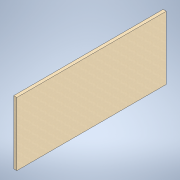
# Autodesk Inventor part: PlatteAußenGross
Saved by Autodesk Inventor 2020.3 (Build 243373000, 373)
## iProperties
Created: 2021-02-12
Part Number: PlatteAußenGross
Material: Generisch
Document SubType Name: Modeling
Designer: Stefan
Density: 1 g/cm^3
Appearance: Pappel
Author: Stefan
Autodesk Inventor part; units mm, degrees
(part 1 of 7)
ref_plane "YZ Plane" through (0, 0, 0) normal (1, 0, 0) x (0, 1, 0)
ref_plane "XZ Plane" through (0, 0, 0) normal (0, 1, 0) x (-1, 0, 0)
ref_plane "XY Plane" through (0, 0, 0) normal (0, 0, 1) x (1, 0, 0)
sketch "Skizze1" plane through (0, 0, 0) normal (1, 0, 0) x (0, 1, 0)
  line L0 (-106.6709, 345.5) -> (93.3291, 345.5)
  line L1 (93.3291, 345.5) -> (93.3291, -126.054)
  line L2 (93.3291, -126.054) -> (-106.6709, -126.054)
  line L3 (-106.6709, -126.054) -> (-106.6709, 345.5)
  point P0 (0, 0)
  dimension "d0" = 200
  dimension "d1" = 471.554
  constraints: 8 end point, 2 parallel, 1 horizontal, 1 perpendicular
  measures "d0" distance of L1.end L2.end
  measures "d1" distance of L0.end L1.end
extrude "Extrusion1" add sketch "Skizze1" along normal blind 10
sketch "Skizze2" plane through (10, 0, 0) normal (1, 0, 0) x (0, 0, -1)
  line L0 (-283.1268, 2.1114) -> (-286.566, 2.1114)
  line L1 (-286.566, 2.1114) -> (-286.566, 4.3601)
  line L2 (-286.566, 4.3601) -> (-286.566, 6.6088)
  line L3 (-286.566, 6.6088) -> (-285.7723, 6.6088)
  line L4 (-285.7723, 6.6088) -> (-285.5154, 6.605)
  line L5 (-285.5154, 6.605) -> (-285.3209, 6.584)
  line L6 (-285.3209, 6.584) -> (-285.1802, 6.5313)
  line L7 (-285.1802, 6.5313) -> (-285.0845, 6.4324)
  line L8 (-285.0845, 6.4324) -> (-285.0252, 6.2729)
  line L9 (-285.0252, 6.2729) -> (-284.9935, 6.0383)
  line L10 (-284.9935, 6.0383) -> (-284.9854, 5.8883)
  line L11 (-284.9854, 5.8883) -> (-284.9809, 5.7142)
  line L12 (-284.9809, 5.7142) -> (-284.9791, 5.514)
  line L13 (-284.9791, 5.514) -> (-284.9787, 5.286)
  line L14 (-284.9787, 5.286) -> (-284.9738, 4.9489)
  line L15 (-284.9738, 4.9489) -> (-284.9586, 4.6676)
  line L16 (-284.9586, 4.6676) -> (-284.9322, 4.4386)
  line L17 (-284.9322, 4.4386) -> (-284.8934, 4.2586)
  line L18 (-284.8934, 4.2586) -> (-284.8415, 4.1244)
  line L19 (-284.8415, 4.1244) -> (-284.7755, 4.0327)
  line L20 (-284.7755, 4.0327) -> (-284.6943, 3.9801)
  line L21 (-284.6943, 3.9801) -> (-284.5971, 3.9632)
  line L22 (-284.5971, 3.9632) -> (-284.5048, 3.9802)
  line L23 (-284.5048, 3.9802) -> (-284.4229, 4.0313)
  line L24 (-284.4229, 4.0313) -> (-284.351, 4.1172)
  line L25 (-284.351, 4.1172) -> (-284.2889, 4.2383)
  line L26 (-284.2889, 4.2383) -> (-284.2364, 4.3954)
  line L27 (-284.2364, 4.3954) -> (-284.1933, 4.589)
  line L28 (-284.1933, 4.589) -> (-284.1592, 4.8195)
  line L29 (-284.1592, 4.8195) -> (-284.1341, 5.0876)
  line L30 (-284.1341, 5.0876) -> (-284.1051, 5.4387)
  line L31 (-284.1051, 5.4387) -> (-284.0699, 5.7083)
  line L32 (-284.0699, 5.7083) -> (-284.02, 5.9069)
  line L33 (-284.02, 5.9069) -> (-283.9472, 6.0453)
  line L34 (-283.9472, 6.0453) -> (-283.843, 6.1343)
  line L35 (-283.843, 6.1343) -> (-283.6992, 6.1846)
  line L36 (-283.6992, 6.1846) -> (-283.5073, 6.2069)
  line L37 (-283.5073, 6.2069) -> (-283.2591, 6.2119)
  line L38 (-283.2591, 6.2119) -> (-283.0108, 6.2069)
  line L39 (-283.0108, 6.2069) -> (-282.819, 6.1846)
  line L40 (-282.819, 6.1846) -> (-282.6752, 6.1343)
  line L41 (-282.6752, 6.1343) -> (-282.571, 6.0453)
  line L42 (-282.571, 6.0453) -> (-282.4982, 5.9069)
  line L43 (-282.4982, 5.9069) -> (-282.4483, 5.7083)
  line L44 (-282.4483, 5.7083) -> (-282.4131, 5.4387)
  line L45 (-282.4131, 5.4387) -> (-282.3841, 5.0876)
  line L46 (-282.3841, 5.0876) -> (-282.359, 4.8195)
  line L47 (-282.359, 4.8195) -> (-282.3249, 4.589)
  line L48 (-282.3249, 4.589) -> (-282.2818, 4.3954)
  line L49 (-282.2818, 4.3954) -> (-282.2293, 4.2383)
  line L50 (-282.2293, 4.2383) -> (-282.1672, 4.1172)
  line L51 (-282.1672, 4.1172) -> (-282.0953, 4.0313)
  line L52 (-282.0953, 4.0313) -> (-282.0134, 3.9802)
  line L53 (-282.0134, 3.9802) -> (-281.9211, 3.9632)
  line L54 (-281.9211, 3.9632) -> (-281.8239, 3.9801)
  line L55 (-281.8239, 3.9801) -> (-281.7427, 4.0327)
  line L56 (-281.7427, 4.0327) -> (-281.6767, 4.1244)
  line L57 (-281.6767, 4.1244) -> (-281.6247, 4.2586)
  line L58 (-281.6247, 4.2586) -> (-281.586, 4.4386)
  line L59 (-281.586, 4.4386) -> (-281.5596, 4.6676)
  line L60 (-281.5596, 4.6676) -> (-281.5444, 4.9489)
  line L61 (-281.5444, 4.9489) -> (-281.5395, 5.286)
  line L62 (-281.5395, 5.286) -> (-281.5395, 6.6088)
  line L63 (-281.5395, 6.6088) -> (-280.6136, 6.6088)
  line L64 (-280.6136, 6.6088) -> (-279.6877, 6.6088)
  line L65 (-279.6877, 6.6088) -> (-279.6877, 4.3601)
  line L66 (-279.6877, 4.3601) -> (-279.6877, 2.1114)
  line L67 (-279.6877, 2.1114) -> (-283.1268, 2.1114)
  line L68 (-282.3332, -54.5023) -> (-284.9787, -54.5023)
  line L69 (-284.9787, -54.5023) -> (-284.9787, -55.4282)
  line L70 (-284.9787, -55.4282) -> (-284.9828, -55.7128)
  line L71 (-284.9828, -55.7128) -> (-284.9999, -55.9325)
  line L72 (-284.9999, -55.9325) -> (-285.0371, -56.0958)
  line L73 (-285.0371, -56.0958) -> (-285.1015, -56.2109)
  line L74 (-285.1015, -56.2109) -> (-285.2001, -56.2859)
  line L75 (-285.2001, -56.2859) -> (-285.3401, -56.3293)
  line L76 (-285.3401, -56.3293) -> (-285.5284, -56.3493)
  line L77 (-285.5284, -56.3493) -> (-285.7723, -56.3542)
  line L78 (-285.7723, -56.3542) -> (-286.566, -56.3542)
  line L79 (-286.566, -56.3542) -> (-286.566, -53.5764)
  line L80 (-286.566, -53.5764) -> (-286.566, -50.7986)
  line L81 (-286.566, -50.7986) -> (-285.7723, -50.7986)
  line L82 (-285.7723, -50.7986) -> (-285.5284, -50.8034)
  line L83 (-285.5284, -50.8034) -> (-285.3401, -50.8234)
  line L84 (-285.3401, -50.8234) -> (-285.2001, -50.8668)
  line L85 (-285.2001, -50.8668) -> (-285.1015, -50.9419)
  line L86 (-285.1015, -50.9419) -> (-285.0371, -51.0569)
  line L87 (-285.0371, -51.0569) -> (-284.9999, -51.2202)
  line L88 (-284.9999, -51.2202) -> (-284.9828, -51.44)
  line L89 (-284.9828, -51.44) -> (-284.9787, -51.7245)
  line L90 (-284.9787, -51.7245) -> (-284.9787, -52.6504)
  line L91 (-284.9787, -52.6504) -> (-282.3332, -52.6504)
  line L92 (-282.3332, -52.6504) -> (-279.6877, -52.6504)
  line L93 (-279.6877, -52.6504) -> (-279.6877, -53.5764)
  line L94 (-279.6877, -53.5764) -> (-279.6877, -54.5023)
  line L95 (-279.6877, -54.5023) -> (-282.3332, -54.5023)
  line L96 (-282.3332, -2.915) -> (-284.9787, -2.915)
  line L97 (-284.9787, -2.915) -> (-284.9787, -3.7087)
  line L98 (-284.9787, -3.7087) -> (-284.9838, -3.9454)
  line L99 (-284.9838, -3.9454) -> (-285.0035, -4.1303)
  line L100 (-285.0035, -4.1303) -> (-285.0438, -4.2698)
  line L101 (-285.0438, -4.2698) -> (-285.1109, -4.3701)
  line L102 (-285.1109, -4.3701) -> (-285.2112, -4.4373)
  line L103 (-285.2112, -4.4373) -> (-285.3507, -4.4775)
  line L104 (-285.3507, -4.4775) -> (-285.5357, -4.4972)
  line L105 (-285.5357, -4.4972) -> (-285.7723, -4.5023)
  line L106 (-285.7723, -4.5023) -> (-286.566, -4.5023)
  line L107 (-286.566, -4.5023) -> (-286.566, -1.8569)
  line L108 (-286.566, -1.8569) -> (-286.566, 0.7887)
  line L109 (-286.566, 0.7887) -> (-285.7723, 0.7887)
  line L110 (-285.7723, 0.7887) -> (-285.5284, 0.7838)
  line L111 (-285.5284, 0.7838) -> (-285.3401, 0.7639)
  line L112 (-285.3401, 0.7639) -> (-285.2001, 0.7204)
  line L113 (-285.2001, 0.7204) -> (-285.1015, 0.6454)
  line L114 (-285.1015, 0.6454) -> (-285.0371, 0.5303)
  line L115 (-285.0371, 0.5303) -> (-284.9999, 0.367)
  line L116 (-284.9999, 0.367) -> (-284.9828, 0.1473)
  line L117 (-284.9828, 0.1473) -> (-284.9787, -0.1373)
  line L118 (-284.9787, -0.1373) -> (-284.9787, -1.0632)
  line L119 (-284.9787, -1.0632) -> (-282.3332, -1.0632)
  line L120 (-282.3332, -1.0632) -> (-279.6877, -1.0632)
  line L121 (-279.6877, -1.0632) -> (-279.6877, -1.9891)
  line L122 (-279.6877, -1.9891) -> (-279.6877, -2.915)
  line L123 (-279.6877, -2.915) -> (-282.3332, -2.915)
  line L124 (-283.1268, -23.2854) -> (-286.566, -23.2854)
  line L125 (-286.566, -23.2854) -> (-286.566, -21.337)
  line L126 (-286.566, -21.337) -> (-286.5595, -20.8821)
  line L127 (-286.5595, -20.8821) -> (-286.5395, -20.4663)
  line L128 (-286.5395, -20.4663) -> (-286.5052, -20.0882)
  line L129 (-286.5052, -20.0882) -> (-286.4555, -19.7464)
  line L130 (-286.4555, -19.7464) -> (-286.3897, -19.4396)
  line L131 (-286.3897, -19.4396) -> (-286.3068, -19.1665)
  line L132 (-286.3068, -19.1665) -> (-286.2059, -18.9258)
  line L133 (-286.2059, -18.9258) -> (-286.0863, -18.7161)
  line L134 (-286.0863, -18.7161) -> (-285.9469, -18.536)
  line L135 (-285.9469, -18.536) -> (-285.7869, -18.3843)
  line L136 (-285.7869, -18.3843) -> (-285.6053, -18.2596)
  line L137 (-285.6053, -18.2596) -> (-285.4014, -18.1606)
  line L138 (-285.4014, -18.1606) -> (-285.1743, -18.0859)
  line L139 (-285.1743, -18.0859) -> (-284.9229, -18.0342)
  line L140 (-284.9229, -18.0342) -> (-284.6465, -18.0041)
  line L141 (-284.6465, -18.0041) -> (-284.3442, -17.9944)
  line L142 (-284.3442, -17.9944) -> (-283.8422, -18.0322)
  line L143 (-283.8422, -18.0322) -> (-283.3938, -18.1451)
  line L144 (-283.3938, -18.1451) -> (-282.9998, -18.3322)
  line L145 (-282.9998, -18.3322) -> (-282.6612, -18.5926)
  line L146 (-282.6612, -18.5926) -> (-282.379, -18.9254)
  line L147 (-282.379, -18.9254) -> (-282.1541, -19.3298)
  line L148 (-282.1541, -19.3298) -> (-281.9874, -19.8047)
  line L149 (-281.9874, -19.8047) -> (-281.8798, -20.3494)
  line L150 (-281.8798, -20.3494) -> (-281.8298, -20.6995)
  line L151 (-281.8298, -20.6995) -> (-281.7777, -20.9648)
  line L152 (-281.7777, -20.9648) -> (-281.7108, -21.157)
  line L153 (-281.7108, -21.157) -> (-281.6165, -21.288)
  line L154 (-281.6165, -21.288) -> (-281.482, -21.3693)
  line L155 (-281.482, -21.3693) -> (-281.2948, -21.4128)
  line L156 (-281.2948, -21.4128) -> (-281.042, -21.4303)
  line L157 (-281.042, -21.4303) -> (-280.711, -21.4336)
  line L158 (-280.711, -21.4336) -> (-280.3819, -21.4365)
  line L159 (-280.3819, -21.4365) -> (-280.1321, -21.4519)
  line L160 (-280.1321, -21.4519) -> (-279.9508, -21.4896)
  line L161 (-279.9508, -21.4896) -> (-279.8269, -21.5595)
  line L162 (-279.8269, -21.5595) -> (-279.7496, -21.6716)
  line L163 (-279.7496, -21.6716) -> (-279.7079, -21.8357)
  line L164 (-279.7079, -21.8357) -> (-279.6909, -22.0617)
  line L165 (-279.6909, -22.0617) -> (-279.6877, -22.3595)
  line L166 (-279.6877, -22.3595) -> (-279.6877, -23.2854)
  line L167 (-279.6877, -23.2854) -> (-283.1268, -23.2854)
  line L168 (-286.9977, -13.047) -> (-287.1591, -13.1536)
  line L169 (-287.1591, -13.1536) -> (-287.3706, -13.2157)
  line L170 (-287.3706, -13.2157) -> (-287.6126, -13.2363)
  line L171 (-287.6126, -13.2363) -> (-287.8655, -13.2182)
  line L172 (-287.8655, -13.2182) -> (-288.1098, -13.1641)
  line L173 (-288.1098, -13.1641) -> (-288.3258, -13.0771)
  line L174 (-288.3258, -13.0771) -> (-288.4939, -12.9598)
  line L175 (-288.4939, -12.9598) -> (-288.5946, -12.8152)
  line L176 (-288.5946, -12.8152) -> (-288.638, -12.5738)
  line L177 (-288.638, -12.5738) -> (-288.5949, -12.338)
  line L178 (-288.5949, -12.338) -> (-288.4815, -12.1216)
  line L179 (-288.4815, -12.1216) -> (-288.3138, -11.9383)
  line L180 (-288.3138, -11.9383) -> (-288.1079, -11.8017)
  line L181 (-288.1079, -11.8017) -> (-287.8797, -11.7257)
  line L182 (-287.8797, -11.7257) -> (-287.6453, -11.724)
  line L183 (-287.6453, -11.724) -> (-287.4208, -11.8103)
  line L184 (-287.4208, -11.8103) -> (-287.2468, -11.942)
  line L185 (-287.2468, -11.942) -> (-287.1022, -12.0954)
  line L186 (-287.1022, -12.0954) -> (-286.9897, -12.263)
  line L187 (-286.9897, -12.263) -> (-286.9117, -12.4371)
  line L188 (-286.9117, -12.4371) -> (-286.8709, -12.6102)
  line L189 (-286.8709, -12.6102) -> (-286.8699, -12.7746)
  line L190 (-286.8699, -12.7746) -> (-286.9113, -12.9227)
  line L191 (-286.9113, -12.9227) -> (-286.9977, -13.047)
  line L192 (-283.1268, -63.2324) -> (-286.566, -63.2324)
  line L193 (-286.566, -63.2324) -> (-286.566, -62.3065)
  line L194 (-286.566, -62.3065) -> (-286.5634, -62.0023)
  line L195 (-286.5634, -62.0023) -> (-286.5465, -61.7733)
  line L196 (-286.5465, -61.7733) -> (-286.5015, -61.6088)
  line L197 (-286.5015, -61.6088) -> (-286.4148, -61.4982)
  line L198 (-286.4148, -61.4982) -> (-286.2726, -61.4307)
  line L199 (-286.2726, -61.4307) -> (-286.0611, -61.3958)
  line L200 (-286.0611, -61.3958) -> (-285.7666, -61.3826)
  line L201 (-285.7666, -61.3826) -> (-285.3755, -61.3806)
  line L202 (-285.3755, -61.3806) -> (-284.9844, -61.3786)
  line L203 (-284.9844, -61.3786) -> (-284.6899, -61.3654)
  line L204 (-284.6899, -61.3654) -> (-284.4784, -61.3305)
  line L205 (-284.4784, -61.3305) -> (-284.3362, -61.263)
  line L206 (-284.3362, -61.263) -> (-284.2495, -61.1524)
  line L207 (-284.2495, -61.1524) -> (-284.2045, -60.9879)
  line L208 (-284.2045, -60.9879) -> (-284.1876, -60.7589)
  line L209 (-284.1876, -60.7589) -> (-284.185, -60.4547)
  line L210 (-284.185, -60.4547) -> (-284.1876, -60.1505)
  line L211 (-284.1876, -60.1505) -> (-284.2045, -59.9214)
  line L212 (-284.2045, -59.9214) -> (-284.2495, -59.757)
  line L213 (-284.2495, -59.757) -> (-284.3362, -59.6463)
  line L214 (-284.3362, -59.6463) -> (-284.4784, -59.5789)
  line L215 (-284.4784, -59.5789) -> (-284.6899, -59.5439)
  line L216 (-284.6899, -59.5439) -> (-284.9844, -59.5308)
  line L217 (-284.9844, -59.5308) -> (-285.3755, -59.5288)
  line L218 (-285.3755, -59.5288) -> (-285.7666, -59.5267)
  line L219 (-285.7666, -59.5267) -> (-286.0611, -59.5136)
  line L220 (-286.0611, -59.5136) -> (-286.2726, -59.4786)
  line L221 (-286.2726, -59.4786) -> (-286.4148, -59.4112)
  line L222 (-286.4148, -59.4112) -> (-286.5015, -59.3005)
  line L223 (-286.5015, -59.3005) -> (-286.5465, -59.1361)
  line L224 (-286.5465, -59.1361) -> (-286.5634, -58.907)
  line L225 (-286.5634, -58.907) -> (-286.566, -58.6028)
  line L226 (-286.566, -58.6028) -> (-286.566, -57.6769)
  line L227 (-286.566, -57.6769) -> (-283.1268, -57.6769)
  line L228 (-283.1268, -57.6769) -> (-279.6877, -57.6769)
  line L229 (-279.6877, -57.6769) -> (-279.6877, -58.6028)
  line L230 (-279.6877, -58.6028) -> (-279.6877, -59.5288)
  line L231 (-279.6877, -59.5288) -> (-281.0104, -59.5288)
  line L232 (-281.0104, -59.5288) -> (-282.3332, -59.5288)
  line L233 (-282.3332, -59.5288) -> (-282.3332, -60.4547)
  line L234 (-282.3332, -60.4547) -> (-282.3332, -61.3806)
  line L235 (-282.3332, -61.3806) -> (-281.0104, -61.3806)
  line L236 (-281.0104, -61.3806) -> (-279.6877, -61.3806)
  line L237 (-279.6877, -61.3806) -> (-279.6877, -62.3065)
  line L238 (-279.6877, -62.3065) -> (-279.6877, -63.2324)
  line L239 (-279.6877, -63.2324) -> (-283.1268, -63.2324)
  line L240 (-279.9599, -15.0165) -> (-280.1469, -15.3533)
  line L241 (-280.1469, -15.3533) -> (-280.4206, -15.6654)
  line L242 (-280.4206, -15.6654) -> (-280.7691, -15.9464)
  line L243 (-280.7691, -15.9464) -> (-281.18, -16.1903)
  line L244 (-281.18, -16.1903) -> (-281.6413, -16.3909)
  line L245 (-281.6413, -16.3909) -> (-282.1409, -16.5419)
  line L246 (-282.1409, -16.5419) -> (-282.6665, -16.6372)
  line L247 (-282.6665, -16.6372) -> (-283.2061, -16.6707)
  line L248 (-283.2061, -16.6707) -> (-283.6182, -16.6579)
  line L249 (-283.6182, -16.6579) -> (-284.0056, -16.6193)
  line L250 (-284.0056, -16.6193) -> (-284.3679, -16.5549)
  line L251 (-284.3679, -16.5549) -> (-284.7049, -16.4649)
  line L252 (-284.7049, -16.4649) -> (-285.0163, -16.3497)
  line L253 (-285.0163, -16.3497) -> (-285.302, -16.2095)
  line L254 (-285.302, -16.2095) -> (-285.5617, -16.0445)
  line L255 (-285.5617, -16.0445) -> (-285.795, -15.8548)
  line L256 (-285.795, -15.8548) -> (-286.0019, -15.6408)
  line L257 (-286.0019, -15.6408) -> (-286.182, -15.4027)
  line L258 (-286.182, -15.4027) -> (-286.335, -15.1406)
  line L259 (-286.335, -15.1406) -> (-286.4608, -14.8549)
  line L260 (-286.4608, -14.8549) -> (-286.559, -14.5456)
  line L261 (-286.559, -14.5456) -> (-286.6295, -14.2132)
  line L262 (-286.6295, -14.2132) -> (-286.672, -13.8578)
  line L263 (-286.672, -13.8578) -> (-286.6862, -13.4796)
  line L264 (-286.6862, -13.4796) -> (-286.6418, -12.95)
  line L265 (-286.6418, -12.95) -> (-286.5142, -12.4623)
  line L266 (-286.5142, -12.4623) -> (-286.3114, -12.0191)
  line L267 (-286.3114, -12.0191) -> (-286.0417, -11.6231)
  line L268 (-286.0417, -11.6231) -> (-285.7133, -11.2768)
  line L269 (-285.7133, -11.2768) -> (-285.3343, -10.9829)
  line L270 (-285.3343, -10.9829) -> (-284.913, -10.7441)
  line L271 (-284.913, -10.7441) -> (-284.4576, -10.563)
  line L272 (-284.4576, -10.563) -> (-283.9761, -10.4421)
  line L273 (-283.9761, -10.4421) -> (-283.4769, -10.3843)
  line L274 (-283.4769, -10.3843) -> (-282.968, -10.3921)
  line L275 (-282.968, -10.3921) -> (-282.4577, -10.4681)
  line L276 (-282.4577, -10.4681) -> (-281.9542, -10.615)
  line L277 (-281.9542, -10.615) -> (-281.4657, -10.8354)
  line L278 (-281.4657, -10.8354) -> (-281.0003, -11.132)
  line L279 (-281.0003, -11.132) -> (-280.5663, -11.5073)
  line L280 (-280.5663, -11.5073) -> (-280.3273, -11.7569)
  line L281 (-280.3273, -11.7569) -> (-280.1338, -11.9853)
  line L282 (-280.1338, -11.9853) -> (-279.9818, -12.2014)
  line L283 (-279.9818, -12.2014) -> (-279.8673, -12.414)
  line L284 (-279.8673, -12.414) -> (-279.7863, -12.6318)
  line L285 (-279.7863, -12.6318) -> (-279.7348, -12.8636)
  line L286 (-279.7348, -12.8636) -> (-279.7089, -13.1182)
  line L287 (-279.7089, -13.1182) -> (-279.7044, -13.4045)
  line L288 (-279.7044, -13.4045) -> (-279.7298, -13.8468)
  line L289 (-279.7298, -13.8468) -> (-279.7864, -14.2982)
  line L290 (-279.7864, -14.2982) -> (-279.8659, -14.7057)
  line L291 (-279.8659, -14.7057) -> (-279.9599, -15.0165)
  line L292 (-284.2512, -19.8948) -> (-284.4701, -19.8746)
  line L293 (-284.4701, -19.8746) -> (-284.6406, -19.8743)
  line L294 (-284.6406, -19.8743) -> (-284.7686, -19.8998)
  line L295 (-284.7686, -19.8998) -> (-284.86, -19.957)
  line L296 (-284.86, -19.957) -> (-284.9208, -20.052)
  line L297 (-284.9208, -20.052) -> (-284.9569, -20.1906)
  line L298 (-284.9569, -20.1906) -> (-284.9742, -20.3787)
  line L299 (-284.9742, -20.3787) -> (-284.9787, -20.6223)
  line L300 (-284.9787, -20.6223) -> (-284.9737, -20.8665)
  line L301 (-284.9737, -20.8665) -> (-284.9544, -21.0566)
  line L302 (-284.9544, -21.0566) -> (-284.9142, -21.1993)
  line L303 (-284.9142, -21.1993) -> (-284.8464, -21.3013)
  line L304 (-284.8464, -21.3013) -> (-284.7444, -21.3691)
  line L305 (-284.7444, -21.3691) -> (-284.6017, -21.4093)
  line L306 (-284.6017, -21.4093) -> (-284.4116, -21.4286)
  line L307 (-284.4116, -21.4286) -> (-284.1675, -21.4336)
  line L308 (-284.1675, -21.4336) -> (-283.9238, -21.4291)
  line L309 (-283.9238, -21.4291) -> (-283.7357, -21.4118)
  line L310 (-283.7357, -21.4118) -> (-283.5971, -21.3757)
  line L311 (-283.5971, -21.3757) -> (-283.5022, -21.3149)
  line L312 (-283.5022, -21.3149) -> (-283.4449, -21.2235)
  line L313 (-283.4449, -21.2235) -> (-283.4194, -21.0955)
  line L314 (-283.4194, -21.0955) -> (-283.4197, -20.925)
  line L315 (-283.4197, -20.925) -> (-283.4399, -20.706)
  line L316 (-283.4399, -20.706) -> (-283.4702, -20.5098)
  line L317 (-283.4702, -20.5098) -> (-283.5141, -20.3475)
  line L318 (-283.5141, -20.3475) -> (-283.5748, -20.2156)
  line L319 (-283.5748, -20.2156) -> (-283.6559, -20.1108)
  line L320 (-283.6559, -20.1108) -> (-283.7607, -20.0297)
  line L321 (-283.7607, -20.0297) -> (-283.8926, -19.969)
  line L322 (-283.8926, -19.969) -> (-284.0549, -19.9251)
  line L323 (-284.0549, -19.9251) -> (-284.2512, -19.8948)
  line L324 (-281.7128, -12.9226) -> (-281.824, -12.8228)
  line L325 (-281.824, -12.8228) -> (-281.9645, -12.7339)
  line L326 (-281.9645, -12.7339) -> (-282.1302, -12.6559)
  line L327 (-282.1302, -12.6559) -> (-282.3167, -12.5893)
  line L328 (-282.3167, -12.5893) -> (-282.7359, -12.4908)
  line L329 (-282.7359, -12.4908) -> (-283.1884, -12.4403)
  line L330 (-283.1884, -12.4403) -> (-283.6408, -12.4398)
  line L331 (-283.6408, -12.4398) -> (-284.0594, -12.491)
  line L332 (-284.0594, -12.491) -> (-284.2456, -12.5366)
  line L333 (-284.2456, -12.5366) -> (-284.4107, -12.5959)
  line L334 (-284.4107, -12.5959) -> (-284.5507, -12.669)
  line L335 (-284.5507, -12.669) -> (-284.6612, -12.7563)
  line L336 (-284.6612, -12.7563) -> (-284.8441, -12.9907)
  line L337 (-284.8441, -12.9907) -> (-284.9548, -13.2466)
  line L338 (-284.9548, -13.2466) -> (-284.996, -13.5123)
  line L339 (-284.996, -13.5123) -> (-284.9703, -13.7763)
  line L340 (-284.9703, -13.7763) -> (-284.8804, -14.0268)
  line L341 (-284.8804, -14.0268) -> (-284.7288, -14.2521)
  line L342 (-284.7288, -14.2521) -> (-284.5182, -14.4408)
  line L343 (-284.5182, -14.4408) -> (-284.2512, -14.581)
  line L344 (-284.2512, -14.581) -> (-283.7927, -14.7007)
  line L345 (-283.7927, -14.7007) -> (-283.3004, -14.7365)
  line L346 (-283.3004, -14.7365) -> (-282.8035, -14.6972)
  line L347 (-282.8035, -14.6972) -> (-282.3313, -14.5917)
  line L348 (-282.3313, -14.5917) -> (-281.9131, -14.4288)
  line L349 (-281.9131, -14.4288) -> (-281.5781, -14.2173)
  line L350 (-281.5781, -14.2173) -> (-281.451, -14.0961)
  line L351 (-281.451, -14.0961) -> (-281.3556, -13.9661)
  line L352 (-281.3556, -13.9661) -> (-281.2957, -13.8283)
  line L353 (-281.2957, -13.8283) -> (-281.275, -13.6839)
  line L354 (-281.275, -13.6839) -> (-281.3095, -13.538)
  line L355 (-281.3095, -13.538) -> (-281.4036, -13.3458)
  line L356 (-281.4036, -13.3458) -> (-281.5428, -13.1324)
  line L357 (-281.5428, -13.1324) -> (-281.7128, -12.9226)
  line L358 (-279.8515, -33.414) -> (-279.9398, -33.4519)
  line L359 (-279.9398, -33.4519) -> (-280.1197, -33.4873)
  line L360 (-280.1197, -33.4873) -> (-280.3801, -33.5194)
  line L361 (-280.3801, -33.5194) -> (-280.7102, -33.5474)
  line L362 (-280.7102, -33.5474) -> (-281.0991, -33.5705)
  line L363 (-281.0991, -33.5705) -> (-281.5359, -33.5879)
  line L364 (-281.5359, -33.5879) -> (-282.0097, -33.599)
  line L365 (-282.0097, -33.599) -> (-282.5095, -33.6029)
  line L366 (-282.5095, -33.6029) -> (-284.9787, -33.6029)
  line L367 (-284.9787, -33.6029) -> (-284.9787, -34.3965)
  line L368 (-284.9787, -34.3965) -> (-284.9838, -34.6331)
  line L369 (-284.9838, -34.6331) -> (-285.0035, -34.8181)
  line L370 (-285.0035, -34.8181) -> (-285.0438, -34.9576)
  line L371 (-285.0438, -34.9576) -> (-285.1109, -35.0579)
  line L372 (-285.1109, -35.0579) -> (-285.2112, -35.125)
  line L373 (-285.2112, -35.125) -> (-285.3507, -35.1653)
  line L374 (-285.3507, -35.1653) -> (-285.5357, -35.185)
  line L375 (-285.5357, -35.185) -> (-285.7723, -35.1901)
  line L376 (-285.7723, -35.1901) -> (-286.566, -35.1901)
  line L377 (-286.566, -35.1901) -> (-286.566, -32.5447)
  line L378 (-286.566, -32.5447) -> (-286.566, -29.8991)
  line L379 (-286.566, -29.8991) -> (-285.7723, -29.8991)
  line L380 (-285.7723, -29.8991) -> (-285.5363, -29.9043)
  line L381 (-285.5363, -29.9043) -> (-285.3516, -29.9239)
  line L382 (-285.3516, -29.9239) -> (-285.2121, -29.964)
  line L383 (-285.2121, -29.964) -> (-285.1118, -30.0306)
  line L384 (-285.1118, -30.0306) -> (-285.0443, -30.1298)
  line L385 (-285.0443, -30.1298) -> (-285.0038, -30.2676)
  line L386 (-285.0038, -30.2676) -> (-284.9839, -30.45)
  line L387 (-284.9839, -30.45) -> (-284.9787, -30.6832)
  line L388 (-284.9787, -30.6832) -> (-284.9787, -31.4673)
  line L389 (-284.9787, -31.4673) -> (-282.3993, -31.543)
  line L390 (-282.3993, -31.543) -> (-279.8199, -31.6187)
  line L391 (-279.8199, -31.6187) -> (-279.7413, -32.4219)
  line L392 (-279.7413, -32.4219) -> (-279.7256, -32.7486)
  line L393 (-279.7256, -32.7486) -> (-279.7412, -33.0446)
  line L394 (-279.7412, -33.0446) -> (-279.7844, -33.2772)
  line L395 (-279.7844, -33.2772) -> (-279.8515, -33.414)
  line L396 (-287.3231, -15.3293) -> (-287.5739, -15.4171)
  line L397 (-287.5739, -15.4171) -> (-287.8298, -15.4272)
  line L398 (-287.8298, -15.4272) -> (-288.0751, -15.3704)
  line L399 (-288.0751, -15.3704) -> (-288.2944, -15.2573)
  line L400 (-288.2944, -15.2573) -> (-288.4719, -15.0986)
  line L401 (-288.4719, -15.0986) -> (-288.5923, -14.9049)
  line L402 (-288.5923, -14.9049) -> (-288.6399, -14.6869)
  line L403 (-288.6399, -14.6869) -> (-288.5991, -14.4552)
  line L404 (-288.5991, -14.4552) -> (-288.4921, -14.2458)
  line L405 (-288.4921, -14.2458) -> (-288.3518, -14.0763)
  line L406 (-288.3518, -14.0763) -> (-288.1854, -13.9492)
  line L407 (-288.1854, -13.9492) -> (-288.0005, -13.8667)
  line L408 (-288.0005, -13.8667) -> (-287.8045, -13.8311)
  line L409 (-287.8045, -13.8311) -> (-287.6048, -13.8447)
  line L410 (-287.6048, -13.8447) -> (-287.4088, -13.9099)
  line L411 (-287.4088, -13.9099) -> (-287.224, -14.0289)
  line L412 (-287.224, -14.0289) -> (-287.0501, -14.1994)
  line L413 (-287.0501, -14.1994) -> (-286.9301, -14.3749)
  line L414 (-286.9301, -14.3749) -> (-286.8635, -14.5519)
  line L415 (-286.8635, -14.5519) -> (-286.8501, -14.7267)
  line L416 (-286.8501, -14.7267) -> (-286.8897, -14.8955)
  line L417 (-286.8897, -14.8955) -> (-286.9819, -15.0546)
  line L418 (-286.9819, -15.0546) -> (-287.1264, -15.2005)
  line L419 (-287.1264, -15.2005) -> (-287.3231, -15.3293)
  line L420 (-283.1268, 8.4606) -> (-286.566, 8.4606)
  line L421 (-286.566, 8.4606) -> (-286.566, 9.3969)
  line L422 (-286.566, 9.3969) -> (-286.5593, 9.699)
  line L423 (-286.5593, 9.699) -> (-286.526, 9.9424)
  line L424 (-286.526, 9.9424) -> (-286.4463, 10.1464)
  line L425 (-286.4463, 10.1464) -> (-286.3002, 10.3302)
  line L426 (-286.3002, 10.3302) -> (-286.1961, 10.4206)
  line L427 (-286.1961, 10.4206) -> (-286.0679, 10.5131)
  line L428 (-286.0679, 10.5131) -> (-285.9133, 10.6102)
  line L429 (-285.9133, 10.6102) -> (-285.7296, 10.7143)
  line L430 (-285.7296, 10.7143) -> (-285.5145, 10.8278)
  line L431 (-285.5145, 10.8278) -> (-285.2654, 10.9531)
  line L432 (-285.2654, 10.9531) -> (-284.9799, 11.0926)
  line L433 (-284.9799, 11.0926) -> (-284.6554, 11.2487)
  line L434 (-284.6554, 11.2487) -> (-282.7449, 12.1643)
  line L435 (-282.7449, 12.1643) -> (-284.6554, 12.1643)
  line L436 (-284.6554, 12.1643) -> (-286.566, 12.1643)
  line L437 (-286.566, 12.1643) -> (-286.566, 13.0981)
  line L438 (-286.566, 13.0981) -> (-286.566, 14.032)
  line L439 (-286.566, 14.032) -> (-283.193, 13.9579)
  line L440 (-283.193, 13.9579) -> (-279.8199, 13.8839)
  line L441 (-279.8199, 13.8839) -> (-279.7416, 12.9556)
  line L442 (-279.7416, 12.9556) -> (-279.7217, 12.6521)
  line L443 (-279.7217, 12.6521) -> (-279.733, 12.4091)
  line L444 (-279.733, 12.4091) -> (-279.7957, 12.2058)
  line L445 (-279.7957, 12.2058) -> (-279.9303, 12.0213)
  line L446 (-279.9303, 12.0213) -> (-280.0309, 11.9295)
  line L447 (-280.0309, 11.9295) -> (-280.1571, 11.8347)
  line L448 (-280.1571, 11.8347) -> (-280.3113, 11.734)
  line L449 (-280.3113, 11.734) -> (-280.4963, 11.6251)
  line L450 (-280.4963, 11.6251) -> (-280.7144, 11.5051)
  line L451 (-280.7144, 11.5051) -> (-280.9683, 11.3716)
  line L452 (-280.9683, 11.3716) -> (-281.2605, 11.2219)
  line L453 (-281.2605, 11.2219) -> (-281.5935, 11.0534)
  line L454 (-281.5935, 11.0534) -> (-283.5237, 10.0794)
  line L455 (-283.5237, 10.0794) -> (-281.6057, 10.0636)
  line L456 (-281.6057, 10.0636) -> (-279.6877, 10.0479)
  line L457 (-279.6877, 10.0479) -> (-279.6877, 9.2542)
  line L458 (-279.6877, 9.2542) -> (-279.6877, 8.4606)
  line L459 (-279.6877, 8.4606) -> (-283.1268, 8.4606)
  line L460 (-283.1161, -49.4759) -> (-286.566, -49.4759)
  line L461 (-286.566, -49.4759) -> (-286.566, -48.5499)
  line L462 (-286.566, -48.5499) -> (-286.566, -47.624)
  line L463 (-286.566, -47.624) -> (-284.0672, -47.624)
  line L464 (-284.0672, -47.624) -> (-281.5685, -47.624)
  line L465 (-281.5685, -47.624) -> (-281.4879, -46.3674)
  line L466 (-281.4879, -46.3674) -> (-281.4593, -45.9683)
  line L467 (-281.4593, -45.9683) -> (-281.4255, -45.664)
  line L468 (-281.4255, -45.664) -> (-281.3775, -45.4416)
  line L469 (-281.3775, -45.4416) -> (-281.3065, -45.2883)
  line L470 (-281.3065, -45.2883) -> (-281.2035, -45.1915)
  line L471 (-281.2035, -45.1915) -> (-281.0596, -45.1381)
  line L472 (-281.0596, -45.1381) -> (-280.866, -45.1155)
  line L473 (-280.866, -45.1155) -> (-280.6136, -45.1108)
  line L474 (-280.6136, -45.1108) -> (-279.8199, -45.1108)
  line L475 (-279.8199, -45.1108) -> (-279.7431, -47.2933)
  line L476 (-279.7431, -47.2933) -> (-279.6663, -49.4759)
  line L477 (-279.6663, -49.4759) -> (-283.1161, -49.4759)
  line L478 (-280.0821, -40.415) -> (-280.2367, -40.7459)
  line L479 (-280.2367, -40.7459) -> (-280.3799, -40.9904)
  line L480 (-280.3799, -40.9904) -> (-280.5189, -41.1502)
  line L481 (-280.5189, -41.1502) -> (-280.6611, -41.2273)
  line L482 (-280.6611, -41.2273) -> (-280.8138, -41.2235)
  line L483 (-280.8138, -41.2235) -> (-280.9843, -41.1406)
  line L484 (-280.9843, -41.1406) -> (-281.18, -40.9803)
  line L485 (-281.18, -40.9803) -> (-281.4082, -40.7446)
  line L486 (-281.4082, -40.7446) -> (-281.5409, -40.5891)
  line L487 (-281.5409, -40.5891) -> (-281.6399, -40.4491)
  line L488 (-281.6399, -40.4491) -> (-281.7061, -40.3177)
  line L489 (-281.7061, -40.3177) -> (-281.7405, -40.1877)
  line L490 (-281.7405, -40.1877) -> (-281.7443, -40.0522)
  line L491 (-281.7443, -40.0522) -> (-281.7184, -39.904)
  line L492 (-281.7184, -39.904) -> (-281.6638, -39.7362)
  line L493 (-281.6638, -39.7362) -> (-281.5815, -39.5417)
  line L494 (-281.5815, -39.5417) -> (-281.4483, -39.2221)
  line L495 (-281.4483, -39.2221) -> (-281.3554, -38.9378)
  line L496 (-281.3554, -38.9378) -> (-281.3028, -38.6911)
  line L497 (-281.3028, -38.6911) -> (-281.2903, -38.4843)
  line L498 (-281.2903, -38.4843) -> (-281.3178, -38.3196)
  line L499 (-281.3178, -38.3196) -> (-281.3853, -38.1992)
  line L500 (-281.3853, -38.1992) -> (-281.4926, -38.1253)
  line L501 (-281.4926, -38.1253) -> (-281.6397, -38.1002)
  line L502 (-281.6397, -38.1002) -> (-281.7199, -38.1177)
  line L503 (-281.7199, -38.1177) -> (-281.8081, -38.168)
  line L504 (-281.8081, -38.168) -> (-281.9014, -38.2476)
  line L505 (-281.9014, -38.2476) -> (-281.997, -38.3528)
  line L506 (-281.997, -38.3528) -> (-282.1833, -38.6262)
  line L507 (-282.1833, -38.6262) -> (-282.3439, -38.96)
  line L508 (-282.3439, -38.96) -> (-282.5403, -39.4002)
  line L509 (-282.5403, -39.4002) -> (-282.7632, -39.7977)
  line L510 (-282.7632, -39.7977) -> (-283.0076, -40.1476)
  line L511 (-283.0076, -40.1476) -> (-283.2686, -40.445)
  line L512 (-283.2686, -40.445) -> (-283.5414, -40.6849)
  line L513 (-283.5414, -40.6849) -> (-283.8209, -40.8623)
  line L514 (-283.8209, -40.8623) -> (-284.1024, -40.9724)
  line L515 (-284.1024, -40.9724) -> (-284.3808, -41.0102)
  line L516 (-284.3808, -41.0102) -> (-284.6802, -40.9915)
  line L517 (-284.6802, -40.9915) -> (-284.9642, -40.9366)
  line L518 (-284.9642, -40.9366) -> (-285.2314, -40.8478)
  line L519 (-285.2314, -40.8478) -> (-285.4806, -40.7272)
  line L520 (-285.4806, -40.7272) -> (-285.7103, -40.5769)
  line L521 (-285.7103, -40.5769) -> (-285.9193, -40.399)
  line L522 (-285.9193, -40.399) -> (-286.106, -40.1956)
  line L523 (-286.106, -40.1956) -> (-286.2693, -39.969)
  line L524 (-286.2693, -39.969) -> (-286.4077, -39.7212)
  line L525 (-286.4077, -39.7212) -> (-286.5198, -39.4543)
  line L526 (-286.5198, -39.4543) -> (-286.6044, -39.1705)
  line L527 (-286.6044, -39.1705) -> (-286.6601, -38.872)
  line L528 (-286.6601, -38.872) -> (-286.6855, -38.5608)
  line L529 (-286.6855, -38.5608) -> (-286.6792, -38.2391)
  line L530 (-286.6792, -38.2391) -> (-286.64, -37.909)
  line L531 (-286.64, -37.909) -> (-286.5664, -37.5726)
  line L532 (-286.5664, -37.5726) -> (-286.4429, -37.1536)
  line L533 (-286.4429, -37.1536) -> (-286.3201, -36.8276)
  line L534 (-286.3201, -36.8276) -> (-286.1919, -36.5898)
  line L535 (-286.1919, -36.5898) -> (-286.0524, -36.4358)
  line L536 (-286.0524, -36.4358) -> (-285.8954, -36.3607)
  line L537 (-285.8954, -36.3607) -> (-285.7151, -36.3601)
  line L538 (-285.7151, -36.3601) -> (-285.5054, -36.4293)
  line L539 (-285.5054, -36.4293) -> (-285.2604, -36.5636)
  line L540 (-285.2604, -36.5636) -> (-285.1148, -36.6648)
  line L541 (-285.1148, -36.6648) -> (-285.0011, -36.7703)
  line L542 (-285.0011, -36.7703) -> (-284.9173, -36.8867)
  line L543 (-284.9173, -36.8867) -> (-284.8617, -37.0205)
  line L544 (-284.8617, -37.0205) -> (-284.8322, -37.1784)
  line L545 (-284.8322, -37.1784) -> (-284.8269, -37.3669)
  line L546 (-284.8269, -37.3669) -> (-284.8439, -37.5926)
  line L547 (-284.8439, -37.5926) -> (-284.8813, -37.8621)
  line L548 (-284.8813, -37.8621) -> (-284.9154, -38.1145)
  line L549 (-284.9154, -38.1145) -> (-284.9326, -38.3347)
  line L550 (-284.9326, -38.3347) -> (-284.9339, -38.5225)
  line L551 (-284.9339, -38.5225) -> (-284.9207, -38.6777)
  line L552 (-284.9207, -38.6777) -> (-284.8939, -38.8003)
  line L553 (-284.8939, -38.8003) -> (-284.8547, -38.89)
  line L554 (-284.8547, -38.89) -> (-284.8044, -38.9468)
  line L555 (-284.8044, -38.9468) -> (-284.7439, -38.9706)
  line L556 (-284.7439, -38.9706) -> (-284.6745, -38.9612)
  line L557 (-284.6745, -38.9612) -> (-284.5973, -38.9185)
  line L558 (-284.5973, -38.9185) -> (-284.5134, -38.8423)
  line L559 (-284.5134, -38.8423) -> (-284.424, -38.7326)
  line L560 (-284.424, -38.7326) -> (-284.3302, -38.5893)
  line L561 (-284.3302, -38.5893) -> (-284.2332, -38.4121)
  line L562 (-284.2332, -38.4121) -> (-284.1341, -38.2009)
  line L563 (-284.1341, -38.2009) -> (-284.034, -37.9557)
  line L564 (-284.034, -37.9557) -> (-283.8781, -37.5853)
  line L565 (-283.8781, -37.5853) -> (-283.7085, -37.2526)
  line L566 (-283.7085, -37.2526) -> (-283.526, -36.9581)
  line L567 (-283.526, -36.9581) -> (-283.3319, -36.7021)
  line L568 (-283.3319, -36.7021) -> (-283.127, -36.4849)
  line L569 (-283.127, -36.4849) -> (-282.9124, -36.3068)
  line L570 (-282.9124, -36.3068) -> (-282.6893, -36.1683)
  line L571 (-282.6893, -36.1683) -> (-282.4584, -36.0697)
  line L572 (-282.4584, -36.0697) -> (-282.221, -36.0113)
  line L573 (-282.221, -36.0113) -> (-281.9781, -35.9934)
  line L574 (-281.9781, -35.9934) -> (-281.7306, -36.0164)
  line L575 (-281.7306, -36.0164) -> (-281.4795, -36.0807)
  line L576 (-281.4795, -36.0807) -> (-281.226, -36.1865)
  line L577 (-281.226, -36.1865) -> (-280.9711, -36.3343)
  line L578 (-280.9711, -36.3343) -> (-280.7157, -36.5244)
  line L579 (-280.7157, -36.5244) -> (-280.461, -36.7571)
  line L580 (-280.461, -36.7571) -> (-280.1654, -37.1072)
  line L581 (-280.1654, -37.1072) -> (-279.9401, -37.4941)
  line L582 (-279.9401, -37.4941) -> (-279.7854, -37.9148)
  line L583 (-279.7854, -37.9148) -> (-279.7016, -38.366)
  line L584 (-279.7016, -38.366) -> (-279.6891, -38.8448)
  line L585 (-279.6891, -38.8448) -> (-279.7481, -39.348)
  line L586 (-279.7481, -39.348) -> (-279.879, -39.8724)
  line L587 (-279.879, -39.8724) -> (-280.0821, -40.415)
  line L588 (-283.1268, -8.7351) -> (-286.566, -8.7351)
  line L589 (-286.566, -8.7351) -> (-286.566, -7.8092)
  line L590 (-286.566, -7.8092) -> (-286.566, -6.8833)
  line L591 (-286.566, -6.8833) -> (-284.0528, -6.8833)
  line L592 (-284.0528, -6.8833) -> (-281.5395, -6.8833)
  line L593 (-281.5395, -6.8833) -> (-281.5395, -5.6928)
  line L594 (-281.5395, -5.6928) -> (-281.5375, -5.3017)
  line L595 (-281.5375, -5.3017) -> (-281.5244, -5.0072)
  line L596 (-281.5244, -5.0072) -> (-281.4894, -4.7957)
  line L597 (-281.4894, -4.7957) -> (-281.422, -4.6535)
  line L598 (-281.422, -4.6535) -> (-281.3113, -4.5668)
  line L599 (-281.3113, -4.5668) -> (-281.1468, -4.5218)
  line L600 (-281.1468, -4.5218) -> (-280.9178, -4.5049)
  line L601 (-280.9178, -4.5049) -> (-280.6136, -4.5023)
  line L602 (-280.6136, -4.5023) -> (-279.6877, -4.5023)
  line L603 (-279.6877, -4.5023) -> (-279.6877, -6.6188)
  line L604 (-279.6877, -6.6188) -> (-279.6877, -8.7351)
  line L605 (-279.6877, -8.7351) -> (-283.1268, -8.7351)
  line L606 (-280.0051, -29.5817) -> (-280.1974, -29.7367)
  line L607 (-280.1974, -29.7367) -> (-280.4048, -29.8367)
  line L608 (-280.4048, -29.8367) -> (-280.6215, -29.8824)
  line L609 (-280.6215, -29.8824) -> (-280.8418, -29.8748)
  line L610 (-280.8418, -29.8748) -> (-281.06, -29.8149)
  line L611 (-281.06, -29.8149) -> (-281.2703, -29.7033)
  line L612 (-281.2703, -29.7033) -> (-281.4669, -29.5411)
  line L613 (-281.4669, -29.5411) -> (-281.6442, -29.3292)
  line L614 (-281.6442, -29.3292) -> (-281.8057, -29.0367)
  line L615 (-281.8057, -29.0367) -> (-281.8798, -28.7555)
  line L616 (-281.8798, -28.7555) -> (-281.8716, -28.494)
  line L617 (-281.8716, -28.494) -> (-281.7858, -28.2608)
  line L618 (-281.7858, -28.2608) -> (-281.6274, -28.0645)
  line L619 (-281.6274, -28.0645) -> (-281.4012, -27.9137)
  line L620 (-281.4012, -27.9137) -> (-281.112, -27.8169)
  line L621 (-281.112, -27.8169) -> (-280.7649, -27.7828)
  line L622 (-280.7649, -27.7828) -> (-280.5839, -27.7952)
  line L623 (-280.5839, -27.7952) -> (-280.4164, -27.8312)
  line L624 (-280.4164, -27.8312) -> (-280.2633, -27.8885)
  line L625 (-280.2633, -27.8885) -> (-280.1256, -27.965)
  line L626 (-280.1256, -27.965) -> (-279.8998, -28.1666)
  line L627 (-279.8998, -28.1666) -> (-279.7465, -28.4186)
  line L628 (-279.7465, -28.4186) -> (-279.6731, -28.7036)
  line L629 (-279.6731, -28.7036) -> (-279.6867, -29.0041)
  line L630 (-279.6867, -29.0041) -> (-279.7286, -29.1547)
  line L631 (-279.7286, -29.1547) -> (-279.795, -29.3026)
  line L632 (-279.795, -29.3026) -> (-279.8868, -29.4457)
  line L633 (-279.8868, -29.4457) -> (-280.0051, -29.5817)
  line L634 (-309.1565, 14.0162) -> (-327.675, 14.0162)
  line L635 (-327.675, 14.0162) -> (-327.675, 23.2754)
  line L636 (-327.675, 23.2754) -> (-327.675, 32.5347)
  line L637 (-327.675, 32.5347) -> (-318.548, 32.5347)
  line L638 (-318.548, 32.5347) -> (-309.421, 32.5347)
  line L639 (-309.421, 32.5347) -> (-309.421, 41.6616)
  line L640 (-309.421, 41.6616) -> (-309.421, 50.7886)
  line L641 (-309.421, 50.7886) -> (-300.0295, 50.7886)
  line L642 (-300.0295, 50.7886) -> (-290.638, 50.7886)
  line L643 (-290.638, 50.7886) -> (-290.638, 32.4024)
  line L644 (-290.638, 32.4024) -> (-290.638, 14.0162)
  line L645 (-290.638, 14.0162) -> (-309.1565, 14.0162)
  line L646 (-309.2888, -24.6081) -> (-327.675, -24.6081)
  line L647 (-327.675, -24.6081) -> (-327.675, -6.2219)
  line L648 (-327.675, -6.2219) -> (-327.675, 12.1643)
  line L649 (-327.675, 12.1643) -> (-318.4158, 12.1643)
  line L650 (-318.4158, 12.1643) -> (-309.1565, 12.1643)
  line L651 (-309.1565, 12.1643) -> (-309.1565, 3.0373)
  line L652 (-309.1565, 3.0373) -> (-309.1565, -6.0896)
  line L653 (-309.1565, -6.0896) -> (-300.0295, -6.0896)
  line L654 (-300.0295, -6.0896) -> (-290.9025, -6.0896)
  line L655 (-290.9025, -6.0896) -> (-290.9025, -15.3489)
  line L656 (-290.9025, -15.3489) -> (-290.9025, -24.6081)
  line L657 (-290.9025, -24.6081) -> (-309.2888, -24.6081)
  line L658 (-309.1531, -63.2324) -> (-327.675, -63.2324)
  line L659 (-327.675, -63.2324) -> (-327.675, -53.9732)
  line L660 (-327.675, -53.9732) -> (-327.675, -44.7139)
  line L661 (-327.675, -44.7139) -> (-323.1811, -44.7139)
  line L662 (-323.1811, -44.7139) -> (-318.6871, -44.7139)
  line L663 (-318.6871, -44.7139) -> (-318.6176, -35.5208)
  line L664 (-318.6176, -35.5208) -> (-318.548, -26.3277)
  line L665 (-318.548, -26.3277) -> (-309.2888, -26.3277)
  line L666 (-309.2888, -26.3277) -> (-300.0295, -26.3277)
  line L667 (-300.0295, -26.3277) -> (-299.96, -35.5146)
  line L668 (-299.96, -35.5146) -> (-299.8904, -44.7015)
  line L669 (-299.8904, -44.7015) -> (-295.3303, -44.7739)
  line L670 (-295.3303, -44.7739) -> (-290.7703, -44.8462)
  line L671 (-290.7703, -44.8462) -> (-290.7007, -54.0393)
  line L672 (-290.7007, -54.0393) -> (-290.6311, -63.2324)
  line L673 (-290.6311, -63.2324) -> (-309.1531, -63.2324)
  line L674 (-266.9776, -42.0774) -> (-267.2374, -42.0809)
  line L675 (-267.2374, -42.0809) -> (-267.4332, -42.1023)
  line L676 (-267.4332, -42.1023) -> (-267.5742, -42.1581)
  line L677 (-267.5742, -42.1581) -> (-267.6693, -42.2649)
  line L678 (-267.6693, -42.2649) -> (-267.7275, -42.4392)
  line L679 (-267.7275, -42.4392) -> (-267.758, -42.6976)
  line L680 (-267.758, -42.6976) -> (-267.7656, -42.8636)
  line L681 (-267.7656, -42.8636) -> (-267.7696, -43.0567)
  line L682 (-267.7696, -43.0567) -> (-267.7712, -43.2791)
  line L683 (-267.7712, -43.2791) -> (-267.7715, -43.5329)
  line L684 (-267.7715, -43.5329) -> (-267.7715, -44.9883)
  line L685 (-267.7715, -44.9883) -> (-270.9469, -44.9883)
  line L686 (-270.9469, -44.9883) -> (-274.1224, -44.9883)
  line L687 (-274.1224, -44.9883) -> (-274.1224, -45.7821)
  line L688 (-274.1224, -45.7821) -> (-274.1224, -46.576)
  line L689 (-274.1224, -46.576) -> (-270.1531, -46.576)
  line L690 (-270.1531, -46.576) -> (-266.1838, -46.576)
  line L691 (-266.1838, -46.576) -> (-266.1838, -44.3267)
  line L692 (-266.1838, -44.3267) -> (-266.1838, -42.0774)
  line L693 (-266.1838, -42.0774) -> (-266.9776, -42.0774)
  line L694 (-268.4539, -11.2872) -> (-268.8433, -11.4849)
  line L695 (-268.8433, -11.4849) -> (-269.3013, -11.6243)
  line L696 (-269.3013, -11.6243) -> (-269.8014, -11.7057)
  line L697 (-269.8014, -11.7057) -> (-270.3169, -11.7294)
  line L698 (-270.3169, -11.7294) -> (-270.8214, -11.6957)
  line L699 (-270.8214, -11.6957) -> (-271.2881, -11.6047)
  line L700 (-271.2881, -11.6047) -> (-271.499, -11.5379)
  line L701 (-271.499, -11.5379) -> (-271.6905, -11.4568)
  line L702 (-271.6905, -11.4568) -> (-271.8593, -11.3616)
  line L703 (-271.8593, -11.3616) -> (-272.002, -11.2523)
  line L704 (-272.002, -11.2523) -> (-272.2357, -10.9788)
  line L705 (-272.2357, -10.9788) -> (-272.4015, -10.6542)
  line L706 (-272.4015, -10.6542) -> (-272.4994, -10.2953)
  line L707 (-272.4994, -10.2953) -> (-272.5297, -9.919)
  line L708 (-272.5297, -9.919) -> (-272.4925, -9.5423)
  line L709 (-272.4925, -9.5423) -> (-272.3879, -9.1819)
  line L710 (-272.3879, -9.1819) -> (-272.2161, -8.8548)
  line L711 (-272.2161, -8.8548) -> (-271.9772, -8.5779)
  line L712 (-271.9772, -8.5779) -> (-271.8212, -8.4592)
  line L713 (-271.8212, -8.4592) -> (-271.636, -8.3567)
  line L714 (-271.636, -8.3567) -> (-271.4258, -8.2702)
  line L715 (-271.4258, -8.2702) -> (-271.1948, -8.1997)
  line L716 (-271.1948, -8.1997) -> (-270.6869, -8.1068)
  line L717 (-270.6869, -8.1068) -> (-270.1453, -8.0778)
  line L718 (-270.1453, -8.0778) -> (-269.6034, -8.1124)
  line L719 (-269.6034, -8.1124) -> (-269.0943, -8.2107)
  line L720 (-269.0943, -8.2107) -> (-268.8624, -8.2836)
  line L721 (-268.8624, -8.2836) -> (-268.6512, -8.3723)
  line L722 (-268.6512, -8.3723) -> (-268.4648, -8.4768)
  line L723 (-268.4648, -8.4768) -> (-268.3073, -8.5971)
  line L724 (-268.3073, -8.5971) -> (-268.0495, -8.8962)
  line L725 (-268.0495, -8.8962) -> (-267.8726, -9.2415)
  line L726 (-267.8726, -9.2415) -> (-267.7755, -9.6152)
  line L727 (-267.7755, -9.6152) -> (-267.7573, -9.9995)
  line L728 (-267.7573, -9.9995) -> (-267.817, -10.3766)
  line L729 (-267.817, -10.3766) -> (-267.9537, -10.7288)
  line L730 (-267.9537, -10.7288) -> (-268.1663, -11.0382)
  line L731 (-268.1663, -11.0382) -> (-268.4539, -11.2872)
  line L732 (-266.9776, -48.4283) -> (-267.7715, -48.4283)
  line L733 (-267.7715, -48.4283) -> (-267.7715, -50.0161)
  line L734 (-267.7715, -50.0161) -> (-267.7715, -51.6038)
  line L735 (-267.7715, -51.6038) -> (-268.6977, -51.6038)
  line L736 (-268.6977, -51.6038) -> (-269.6238, -51.6038)
  line L737 (-269.6238, -51.6038) -> (-269.6238, -50.2807)
  line L738 (-269.6238, -50.2807) -> (-269.6269, -49.8693)
  line L739 (-269.6269, -49.8693) -> (-269.6404, -49.553)
  line L740 (-269.6404, -49.553) -> (-269.6703, -49.3194)
  line L741 (-269.6703, -49.3194) -> (-269.7231, -49.156)
  line L742 (-269.7231, -49.156) -> (-269.8047, -49.0506)
  line L743 (-269.8047, -49.0506) -> (-269.9215, -48.9906)
  line L744 (-269.9215, -48.9906) -> (-270.0797, -48.9638)
  line L745 (-270.0797, -48.9638) -> (-270.2854, -48.9576)
  line L746 (-270.2854, -48.9576) -> (-270.4911, -48.9638)
  line L747 (-270.4911, -48.9638) -> (-270.6492, -48.9906)
  line L748 (-270.6492, -48.9906) -> (-270.766, -49.0506)
  line L749 (-270.766, -49.0506) -> (-270.8477, -49.156)
  line L750 (-270.8477, -49.156) -> (-270.9004, -49.3194)
  line L751 (-270.9004, -49.3194) -> (-270.9304, -49.553)
  line L752 (-270.9304, -49.553) -> (-270.9438, -49.8693)
  line L753 (-270.9438, -49.8693) -> (-270.9469, -50.2807)
  line L754 (-270.9469, -50.2807) -> (-270.9473, -50.5087)
  line L755 (-270.9473, -50.5087) -> (-270.9492, -50.709)
  line L756 (-270.9492, -50.709) -> (-270.9537, -50.8832)
  line L757 (-270.9537, -50.8832) -> (-270.9618, -51.0332)
  line L758 (-270.9618, -51.0332) -> (-270.9935, -51.2678)
  line L759 (-270.9935, -51.2678) -> (-271.0528, -51.4274)
  line L760 (-271.0528, -51.4274) -> (-271.1485, -51.5262)
  line L761 (-271.1485, -51.5262) -> (-271.2893, -51.579)
  line L762 (-271.2893, -51.579) -> (-271.4838, -51.6)
  line L763 (-271.4838, -51.6) -> (-271.7408, -51.6038)
  line L764 (-271.7408, -51.6038) -> (-272.5347, -51.6038)
  line L765 (-272.5347, -51.6038) -> (-272.5347, -50.0161)
  line L766 (-272.5347, -50.0161) -> (-272.5347, -48.4283)
  line L767 (-272.5347, -48.4283) -> (-273.3285, -48.4283)
  line L768 (-273.3285, -48.4283) -> (-274.1224, -48.4283)
  line L769 (-274.1224, -48.4283) -> (-274.1224, -50.6776)
  line L770 (-274.1224, -50.6776) -> (-274.1224, -52.9269)
  line L771 (-274.1224, -52.9269) -> (-270.1531, -52.9269)
  line L772 (-270.1531, -52.9269) -> (-266.1838, -52.9269)
  line L773 (-266.1838, -52.9269) -> (-266.1838, -50.6776)
  line L774 (-266.1838, -50.6776) -> (-266.1838, -48.4283)
  line L775 (-266.1838, -48.4283) -> (-266.9776, -48.4283)
  line L776 (-266.9776, -35.7266) -> (-267.7715, -35.7266)
  line L777 (-267.7715, -35.7266) -> (-267.7715, -37.3143)
  line L778 (-267.7715, -37.3143) -> (-267.7715, -38.902)
  line L779 (-267.7715, -38.902) -> (-268.6977, -38.902)
  line L780 (-268.6977, -38.902) -> (-269.6238, -38.902)
  line L781 (-269.6238, -38.902) -> (-269.6238, -37.5789)
  line L782 (-269.6238, -37.5789) -> (-269.6269, -37.1675)
  line L783 (-269.6269, -37.1675) -> (-269.6404, -36.8512)
  line L784 (-269.6404, -36.8512) -> (-269.6703, -36.6176)
  line L785 (-269.6703, -36.6176) -> (-269.7231, -36.4543)
  line L786 (-269.7231, -36.4543) -> (-269.8047, -36.3488)
  line L787 (-269.8047, -36.3488) -> (-269.9215, -36.2889)
  line L788 (-269.9215, -36.2889) -> (-270.0797, -36.262)
  line L789 (-270.0797, -36.262) -> (-270.2854, -36.2558)
  line L790 (-270.2854, -36.2558) -> (-270.4911, -36.262)
  line L791 (-270.4911, -36.262) -> (-270.6492, -36.2889)
  line L792 (-270.6492, -36.2889) -> (-270.766, -36.3488)
  line L793 (-270.766, -36.3488) -> (-270.8477, -36.4543)
  line L794 (-270.8477, -36.4543) -> (-270.9004, -36.6176)
  line L795 (-270.9004, -36.6176) -> (-270.9304, -36.8512)
  line L796 (-270.9304, -36.8512) -> (-270.9438, -37.1675)
  line L797 (-270.9438, -37.1675) -> (-270.9469, -37.5789)
  line L798 (-270.9469, -37.5789) -> (-270.9473, -37.807)
  line L799 (-270.9473, -37.807) -> (-270.9492, -38.0072)
  line L800 (-270.9492, -38.0072) -> (-270.9537, -38.1814)
  line L801 (-270.9537, -38.1814) -> (-270.9618, -38.3314)
  line L802 (-270.9618, -38.3314) -> (-270.9935, -38.5661)
  line L803 (-270.9935, -38.5661) -> (-271.0528, -38.7256)
  line L804 (-271.0528, -38.7256) -> (-271.1485, -38.8245)
  line L805 (-271.1485, -38.8245) -> (-271.2893, -38.8772)
  line L806 (-271.2893, -38.8772) -> (-271.4838, -38.8982)
  line L807 (-271.4838, -38.8982) -> (-271.7408, -38.902)
  line L808 (-271.7408, -38.902) -> (-272.5347, -38.902)
  line L809 (-272.5347, -38.902) -> (-272.5347, -37.3143)
  line L810 (-272.5347, -37.3143) -> (-272.5347, -35.7266)
  line L811 (-272.5347, -35.7266) -> (-273.3285, -35.7266)
  line L812 (-273.3285, -35.7266) -> (-274.1224, -35.7266)
  line L813 (-274.1224, -35.7266) -> (-274.1224, -37.9758)
  line L814 (-274.1224, -37.9758) -> (-274.1224, -40.2251)
  line L815 (-274.1224, -40.2251) -> (-270.1531, -40.2251)
  line L816 (-270.1531, -40.2251) -> (-266.1838, -40.2251)
  line L817 (-266.1838, -40.2251) -> (-266.1838, -37.9758)
  line L818 (-266.1838, -37.9758) -> (-266.1838, -35.7266)
  line L819 (-266.1838, -35.7266) -> (-266.9776, -35.7266)
  line L820 (-266.5648, -8.6003) -> (-266.8005, -8.1443)
  line L821 (-266.8005, -8.1443) -> (-267.1014, -7.7458)
  line L822 (-267.1014, -7.7458) -> (-267.4659, -7.406)
  line L823 (-267.4659, -7.406) -> (-267.8922, -7.1257)
  line L824 (-267.8922, -7.1257) -> (-268.3785, -6.906)
  line L825 (-268.3785, -6.906) -> (-268.9231, -6.7477)
  line L826 (-268.9231, -6.7477) -> (-269.5242, -6.6518)
  line L827 (-269.5242, -6.6518) -> (-270.1801, -6.6194)
  line L828 (-270.1801, -6.6194) -> (-270.8459, -6.6542)
  line L829 (-270.8459, -6.6542) -> (-271.4535, -6.7592)
  line L830 (-271.4535, -6.7592) -> (-272.0019, -6.9339)
  line L831 (-272.0019, -6.9339) -> (-272.4905, -7.1778)
  line L832 (-272.4905, -7.1778) -> (-272.9183, -7.4905)
  line L833 (-272.9183, -7.4905) -> (-273.2847, -7.8715)
  line L834 (-273.2847, -7.8715) -> (-273.5887, -8.3202)
  line L835 (-273.5887, -8.3202) -> (-273.8297, -8.8362)
  line L836 (-273.8297, -8.8362) -> (-273.9789, -9.3616)
  line L837 (-273.9789, -9.3616) -> (-274.0335, -9.8926)
  line L838 (-274.0335, -9.8926) -> (-273.9967, -10.419)
  line L839 (-273.9967, -10.419) -> (-273.8721, -10.9307)
  line L840 (-273.8721, -10.9307) -> (-273.6629, -11.4178)
  line L841 (-273.6629, -11.4178) -> (-273.3725, -11.87)
  line L842 (-273.3725, -11.87) -> (-273.0043, -12.2774)
  line L843 (-273.0043, -12.2774) -> (-272.5617, -12.6298)
  line L844 (-272.5617, -12.6298) -> (-272.2013, -12.84)